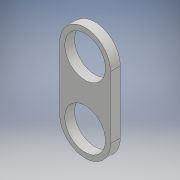
# Autodesk Inventor part: support_axe
Saved by Autodesk Inventor 2018 (Build 220112000, 112)
## iProperties
Created: 2018-02-11
Part Number: support_axe
Material: Générique
Document SubType Name: Modeling
Designer: Tristan
Density: 1 g/cm^3
Appearance: Par défaut
Author: Tristan
Autodesk Inventor part; units mm, degrees
ref_plane "YZ Plane" through (0, 0, 0) normal (1, 0, 0) x (0, 1, 0)
ref_plane "XZ Plane" through (0, 0, 0) normal (0, 1, 0) x (-1, 0, 0)
ref_plane "XY Plane" through (0, 0, 0) normal (0, 0, 1) x (1, 0, 0)
sketch "Esquisse1" plane through (0, 0, 0) normal (0, 1, 0) x (-1, 0, 0)
  arc A0 (13, 0) -> (-13, 0) centre (0, 0) ccw
  arc A1 (-13, -32) -> (13, -32) centre (0, -32) ccw
  line L0 (13, -32) -> (13, 0)
  line L1 (-13, 0) -> (-13, -32)
  circle A2 centre (0, 0) radius 10.4
  circle A3 centre (0, -32) radius 10.4
  line L2 (13, 0) -> (10.4, 0)
  dimension "d4" = 20.8
  dimension "d0" = 26
  dimension "d1" = 26
  dimension "d2" = 26
  dimension "d3" = 32
  dimension "d5" = 20.8
  constraints: 6 end point, 4 point on circle, 3 centre point, 3 coincident, 1 horizontal alignment, 1 parallel, 2 other
  measures "d0" diameter of A0
  measures "d1" diameter of A1
  measures "d2" distance of L1.end L0.start
  measures "d3" distance of L0.start L0.end
  measures "d5" diameter of A3
extrude "Extrusion1" add sketch "Esquisse1" along normal blind 5
